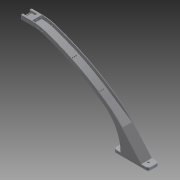
# Autodesk Inventor part: Lickport_Holder _v3
Saved by Autodesk Inventor 2012 SP2 (Build 160219200, 219)
## iProperties
Created: 2015-03-09
Part Number: Lickport_Holder _v3
Material: Default
Document SubType Name: Modeling
Designer: zhaox11
Density: 1 g/cm^3
Author: zhaox11
Autodesk Inventor part; units mm, degrees
ref_plane "YZ Plane" through (0, 0, 0) normal (1, 0, 0) x (0, 1, 0)
ref_plane "XZ Plane" through (0, 0, 0) normal (0, 1, 0) x (-1, 0, 0)
sketch "Sketch1" plane through (0, 0, 0) normal (0, 0, 1) x (1, 0, 0)
  line L0 (-50.8, 9.525) -> (-25.4, 9.525)
  line L1 (-25.4, 9.525) -> (-25.4, 0)
  line L2 (-25.4, 0) -> (-50.8, 0)
  line L3 (-50.8, 0) -> (-50.8, 9.525)
  line L4 (-25.4, -92.075) -> (11.1056, 20.2776)
  arc A0 (5.9961, 4.5523) -> (-25.4, 9.525) centre (-25.4, -92.075) ccw
  arc A1 (3.0527, -4.5065) -> (-25.4, 0) centre (-25.4, -92.075) ccw
  line L5 (-25.4, -92.075) -> (-197.4001, -621.4369)
  line L6 (-158.1658, -500.6861) -> (150.3246, -68.1948)
  arc A2 (150.3246, -68.1948) -> (5.9961, 4.5523) centre (-158.1658, -500.6861) ccw
  line L7 (150.3246, -68.1948) -> (159.8241, -54.8769)
  arc A3 (144.7934, -75.9493) -> (3.0527, -4.5065) centre (-158.1658, -500.6861) ccw
  line L8 (150.3246, -68.1948) -> (144.7934, -75.9493)
  line L9 (307.5871, -155.575) -> (-197.4001, -155.575)
  arc A4 (223.3152, -155.575) -> (150.3246, -68.1948) centre (19.4204, -251.7174) ccw
  arc A5 (212.7322, -155.575) -> (144.7934, -75.9493) centre (19.4204, -251.7174) ccw
  arc A6 (185.8036, -155.575) -> (144.7934, -75.9493) centre (87.9975, -155.575) ccw
  line L10 (87.9975, -155.575) -> (238.9402, -77.834)
  line L11 (189.2177, -103.4429) -> (19.4204, -251.7174)
  line L12 (189.2177, -103.4429) -> (234.7417, -155.575)
  line L13 (185.8036, -155.575) -> (212.7322, -155.575)
  line L14 (223.3152, -155.575) -> (212.7322, -155.575)
  line L15 (223.3152, -155.575) -> (234.7417, -155.575)
  line L16 (150.3246, -68.1948) -> (175.5181, -86.165)
  line L17 (145.7153, -74.6569) -> (144.7934, -75.9493)
  line L18 (144.7934, -75.9493) -> (145.7153, -74.6569)
  line L19 (145.7153, -74.6569) -> (189.2177, -103.4429)
  line L20 (234.7417, -155.575) -> (212.7322, -155.575)
  arc A7 (187.3911, -155.575) -> (145.7153, -74.6569) centre (87.9975, -155.575) ccw
  line L21 (187.3911, -155.575) -> (234.7417, -155.575)
  line L22 (145.7153, -74.6569) -> (150.3246, -68.1948)
  line L23 (234.7417, -155.575) -> (252.6778, -176.1147)
  point P0 (0, 0)
  dimension "d0" = 0
  dimension "d1" = 25.4
  dimension "d2" = 25.4
  dimension "d3" = 9.525
  dimension "d5" = 101.6
  dimension "d6" = 0
  dimension "d7" = 18
  dimension "d8" = 107.3658
  dimension "d29" = 17.5
  dimension "d55" = 165.1
  dimension "d56" = 54.5
  dimension "d57" = 27.25
  dimension "d70" = 7.9375
  constraints: 48 end point, 17 point on circle, 13 point on line, 10 collinear, 9 coincident, 8 centre point, 5 perpendicular, 2 parallel, 1 horizontal
  measures "d0" distance from line of point (0, 0) L2
  measures "d1" distance of L0.start L0.end
  measures "d2" distance from line of point (0, 0) L1
  measures "d3" distance of L2.end L0.start
  measures "d5" distance from line of L0 L4.start
  measures "d6" distance from line of L4.start L1
  measures "d7" angle of L4 L1
  measures "d8" distance from line of point (-158.166, -500.686) L3
  measures "d29" angle of L6 L5
  measures "d55" distance between parallel lines of L9 L0
  measures "d56" angle of L9 L6
  measures "d57" angle of L10 L6
  measures "d70" distance from line of L16 L17.start
extrude "Extrusion9" add sketch "Sketch1" against normal blind 25.4 contours L0 L1 L2 L3 | A0 L4 A1 L1 | A2 L6 A3 L4 | A4 L19 L6 | L6 A7 A5 | A5 A7 L10 A6 | L19 L10 A5 A7 | L12 L9 A4 | L11 A5 L10 | A4 L9 A5 L11 | A5 L10 A7 | L10 A7 L11 A6 | A5 L11 A7 L10 | A5 L9 A7 L11 | L11 A7 L9 A6
sketch "Sketch8" plane through (0, 0, 0) normal (0, 0, 1) x (1, 0, 0)
  line L0 (234.7417, -155.575) -> (185.8036, -155.575)
  line L1 (185.8036, -155.575) -> (185.8036, -161.925)
  line L2 (185.8036, -161.925) -> (234.7417, -161.925)
  line L3 (234.7417, -161.925) -> (234.7417, -155.575)
  point P0 (0, 0)
  dimension "d61" = 6.35
  constraints: 8 end point, 2 parallel, 1 horizontal, 1 perpendicular
  measures "d61" distance of L0.end L1.end
extrude "Extrusion10" add sketch "Sketch8" against normal blind 25.4
sketch "Sketch9" plane through (-50.8, 0, 0) normal (-1, 0, 0) x (0, 0, 1)
  line L0 (-25.4, 9.525) -> (-25.4, 0) projected
  line L1 (0, 0) -> (-25.4, 0) projected
  line L2 (0, 9.525) -> (0, 0) projected
  line L3 (0, 9.525) -> (-25.4, 9.525) projected
  line L4 (-23.8125, 9.525) -> (-1.5875, 9.525)
  line L5 (-1.5875, 9.525) -> (-1.5875, 1.5875)
  line L6 (-1.5875, 1.5875) -> (-23.8125, 1.5875)
  line L7 (-23.8125, 1.5875) -> (-23.8125, 9.525)
  dimension "d64" = 1.5875
  dimension "d65" = 1.5875
  dimension "d66" = 1.5875
  constraints: 8 end point, 2 parallel, 1 horizontal, 1 perpendicular, 1 point on line
  measures "d64" distance between parallel lines of L1 L6
  measures "d65" distance between parallel lines of L2 L5
  measures "d66" distance between parallel lines of L0 L7
sketch3d "3D Sketch2"
  line L0 (-50.8, 9.525, 0) -> (-25.4, 9.525, 0)
  arc A0 (-25.4, 9.525, 0) -> (5.9961, 4.5523, 0) centre (-25.4, -92.075, 0) ccw
  arc A1 (5.9961, 4.5523, 0) -> (150.3246, -68.1948, 0) centre (-158.1658, -500.6861, 0) ccw
  arc A2 (150.3246, -68.1948, 0) -> (189.2177, -103.4429, 0) centre (19.4204, -251.7174, 0) ccw
  line L1 (189.2177, -103.4429, 0) -> (234.7417, -155.575, 0)
sweep "Sweep2" cut profiles "Sketch9" path "3D Sketch2" contours L3 L5 L6 L7
sketch "Sketch13" plane through (228.7629, -160.7959, -1.5875) normal (-0.6577551, 0.7532319, 0) x (0.7532319, 0.6577551, 0)
  line L0 (0, 22.225) -> (0, 0) projected
  line L1 (0, 0) -> (7.9375, 0) projected
  line L2 (0, 22.225) -> (7.9375, 22.225)
  line L3 (7.9375, 22.225) -> (7.9375, 0)
  line L4 (7.9375, 0) -> (0, 0)
  line L5 (0, 0) -> (0, 22.225)
  point P0 (-66.5472, -1.5875)
  constraints: 8 end point, 2 parallel, 1 horizontal, 1 perpendicular
extrude "Extrusion14" cut sketch "Sketch13" against normal blind 25.4
extrude "Extrusion15" add sketch "Sketch1" against normal blind 25.4 contours L19 L10 A5 A7 | L12 L9 A4 | L11 A5 L10 | A4 L9 A5 L11 | A5 L10 A7 | A5 L11 A7 L10 | A5 L9 A7 L11
sketch "Sketch14" plane through (224.2038, -155.575, -1.5875) normal (0, -1, 0) x (1, 0, 0)
  line L0 (0, 0) -> (10.5379, 0)
  line L1 (10.5379, 0) -> (10.5379, -22.225)
  line L2 (10.5379, -22.225) -> (0, -22.225)
  line L3 (0, -22.225) -> (0, 0)
  point P0 (-224.2038, 1.5875)
  constraints: 8 end point, 2 parallel, 1 horizontal, 1 perpendicular
extrude "Extrusion16" add sketch "Sketch14" along normal blind 6.35
sketch "Sketch17" plane through (-50.8, 1.5875, -1.5875) normal (0, 1, 0) x (1, 0, 0)
  line L0 (0, 0) -> (25.4, 0) projected
  line L1 (25.4, 22.225) -> (17.78, 22.225)
  line L2 (17.78, 22.225) -> (17.78, 0)
  line L3 (17.78, 0) -> (25.4, 0)
  line L4 (25.4, 0) -> (25.4, 22.225)
  point P0 (50.8, -1.5875)
  dimension "d99" = 7.62
  constraints: 8 end point, 2 parallel, 1 horizontal, 1 perpendicular, 1 point on line
  measures "d99" distance of L1.start L1.end
extrude "Extrusion19" add sketch "Sketch17" along normal blind 7.9375
sketch "Sketch19" plane through (-25.4, 1.5875, -1.5875) normal (1, 0, 0) x (0, 0, -1)
  line L0 (22.225, 7.9375) -> (0, 7.9375) projected
  line L1 (22.225, 0) -> (0, 0) projected
  circle A0 centre (11.1125, 4.3942) radius 1.143
  line L2 (23.8125, 7.9375) -> (23.8125, 2.9648) projected
  circle A1 centre (11.1125, 1.143) radius 1.143
  circle A2 centre (1.143, 4.3942) radius 1.143
  circle A3 centre (21.082, 4.3942) radius 1.143
  line L3 (0, 7.9375) -> (0, 2.9648) projected
  line L4 (22.225, 2.9648) -> (22.225, 7.9375) projected
  line L5 (22.225, 7.9375) -> (22.225, 0) projected
  line L6 (21.082, 5.5372) -> (21.082, 4.3942)
  point P0 (-1.5875, -1.5875)
  dimension "d109" = 2.286
  dimension "d102" = 2.286
  dimension "d103" = 4.3942
  dimension "d104" = 7.9375
  dimension "d106" = 12.7
  dimension "d107" = 2.286
  dimension "d108" = 2.286
  dimension "d110" = 4.3942
  dimension "d111" = 4.3942
  dimension "d127" = 2.4003
  constraints: 3 centre point, 2 end point, 2 tangent, 1 coincident, 1 parallel, 1 vertical, 1 vertical alignment, 2 other
  measures "d102" diameter of A0
  measures "d103" distance from line of L1 A0.centre
  measures "d104" distance between parallel lines of L1 L0
  measures "d106" distance from line of L2 A0.centre
  measures "d107" diameter of A1
  measures "d108" diameter of A2
  measures "d110" distance from line of L1 A2.centre
  measures "d111" distance from line of L1 L6.end
  measures "d127" distance from line of L6.start L0
extrude "Extrusion20" cut sketch "Sketch19" against normal blind 7.62
sketch "Sketch20" plane through (-50.8, 1.5875, -1.5875) normal (0, 1, 0) x (1, 0, 0)
  line L0 (0, 0) -> (17.78, 0) projected
  line L1 (0, 22.225) -> (1.5875, 22.225)
  line L2 (1.5875, 22.225) -> (1.5875, 0)
  line L3 (1.5875, 0) -> (0, 0)
  line L4 (0, 0) -> (0, 22.225)
  point P0 (50.8, -1.5875)
  dimension "d114" = 1.5875
  constraints: 8 end point, 2 parallel, 1 horizontal, 1 perpendicular, 1 point on line
  measures "d114" distance between parallel lines of L2 L4
extrude "Extrusion21" add sketch "Sketch20" along normal blind 1.5875
sketch "Sketch21" plane through (-50.8, 3.175, -1.5875) normal (0, 1, 0) x (1, 0, 0)
  line L0 (1.5875, 22.225) -> (1.5875, 0) projected
  line L1 (0, 22.225) -> (1.5875, 22.225)
  line L2 (1.5875, 22.225) -> (1.5875, 19.05)
  line L3 (1.5875, 19.05) -> (0, 19.05)
  line L4 (0, 19.05) -> (0, 22.225)
  line L5 (0, 0) -> (1.5875, 0)
  line L6 (1.5875, 0) -> (1.5875, 3.175)
  line L7 (1.5875, 3.175) -> (0, 3.175)
  line L8 (0, 3.175) -> (0, 0)
  point P0 (50.8, -1.5875)
  dimension "d117" = 3.175
  dimension "d118" = 3.175
  constraints: 16 end point, 4 parallel, 2 horizontal, 2 perpendicular, 2 point on line
  measures "d117" distance of L3.end L1.start
  measures "d118" distance of L7.end L5.start
extrude "Extrusion22" add sketch "Sketch21" along normal blind 6.35
sketch "Sketch22" plane through (-33.02, 1.5875, -23.8125) normal (0, 0, 1) x (1, 0, 0)
  line L0 (0, 4.3942) -> (0, 7.9375) projected
  line L1 (-16.1925, 7.9375) -> (0, 7.9375) projected
  line L2 (-16.1925, 7.9375) -> (0, 7.9375)
  line L3 (0, 7.9375) -> (0, 6.35)
  line L4 (0, 6.35) -> (-16.1925, 6.35)
  line L5 (-16.1925, 6.35) -> (-16.1925, 7.9375)
  point P0 (33.02, -1.5875)
  dimension "d121" = 1.5875
  constraints: 8 end point, 2 parallel, 1 horizontal, 1 perpendicular, 1 point on line
  measures "d121" distance between parallel lines of L4 L2
extrude "Extrusion23" add sketch "Sketch22" along normal blind 3.175
sketch "Sketch23" plane through (-33.02, 5.9817, -1.5875) normal (0, 0, -1) x (-1, 0, 0)
  line L0 (16.1925, -4.3942) -> (16.1925, 3.5433) projected
  line L1 (0, 3.5433) -> (16.1925, 3.5433)
  line L2 (16.1925, 3.5433) -> (16.1925, 1.9558)
  line L3 (16.1925, 1.9558) -> (0, 1.9558)
  line L4 (0, 1.9558) -> (0, 3.5433)
  point P0 (-33.02, -5.9817)
  dimension "d124" = 1.5875
  constraints: 8 end point, 2 parallel, 1 horizontal, 1 perpendicular, 1 point on line
  measures "d124" distance between parallel lines of L3 L1
extrude "Extrusion24" add sketch "Sketch23" along normal blind 3.175
sketch "Sketch24" plane through (0, 0, 0) normal (0, 0, 1) x (1, 0, 0)
  circle A0 centre (-10.4817, 2.1152) radius 1.27
  arc A1 (5.9961, 4.5523) -> (-25.4, 9.525) centre (-25.4, -92.075) ccw projected
  line L0 (-50.8, 0) -> (-25.4, 0) projected
  arc A2 (3.0527, -4.5065) -> (-25.4, 0) centre (-25.4, -92.075) ccw projected
  line L1 (234.7417, -161.925) -> (234.7417, -155.575) projected
  line L2 (-25.4, -92.075) -> (-7.073, 23.6369)
  line L3 (-25.4, -92.075) -> (-25.4, 0)
  line L4 (-10.4817, 2.1152) -> (-5.7845, 1.3712)
  line L5 (-25.4, -92.075) -> (-0.7179, 0.0398)
  line L6 (-0.7179, 0.0398) -> (6.1959, -1.8127)
  circle A3 centre (-0.7179, 0.0398) radius 1.27
  point P0 (0, 0)
  dimension "d128" = 2.54
  dimension "d134" = 9
  dimension "d135" = 92.075
  dimension "d136" = 95.3643
  dimension "d137" = 14.9183
  dimension "d138" = 2.1152
  dimension "d139" = 6
  dimension "d140" = 95.3643
  dimension "d141" = 2.54
  constraints: 10 end point, 2 centre point, 2 coincident, 2 perpendicular, 1 parallel, 1 point on line
  measures "d128" diameter of A0
  measures "d134" angle of L2 L3
  measures "d135" distance of L2.start L0.end
  measures "d136" distance from line of A1.centre L4
  measures "d137" distance from line of L3 A0.centre
  measures "d138" distance from line of L0 A0.centre
  measures "d139" angle of L5 L2
  measures "d140" distance from line of A1.centre L6
  measures "d141" diameter of A3
extrude "Extrusion26" cut sketch "Sketch24" against normal blind 25.4 contours A0 L4 L2 | L2 A0 | A0 L2 L4 | A3 L6 L5 | L5 L6 A3
sketch "Sketch25" plane through (185.8036, -161.925, 0) normal (-1, 0, 0) x (0, 0, 1)
  line L0 (-25.4, 6.35) -> (-25.4, 0) projected
  line L1 (0, 0) -> (-25.4, 0) projected
  line L2 (-25.4, 6.35) -> (0, 6.35)
  line L3 (0, 6.35) -> (0, 0)
  line L4 (0, 0) -> (-25.4, 0)
  line L5 (-25.4, 0) -> (-25.4, 6.35)
  point P0 (0, 161.925)
  constraints: 8 end point, 2 parallel, 1 horizontal, 1 perpendicular
extrude "Extrusion27" add sketch "Sketch25" along normal blind 16.51
sketch "Sketch26" plane through (234.7417, -161.925, -25.4) normal (0, -1, 0) x (1, 0, 0)
  line L0 (0, 25.4) -> (0, 0) projected
  line L1 (-65.4481, 25.4) -> (0, 25.4) projected
  line L2 (-65.4481, 25.4) -> (-65.4481, 0) projected
  line L3 (-65.4481, 0) -> (0, 0) projected
  line L4 (-65.4481, 25.4) -> (17.1019, 25.4)
  line L5 (17.1019, 25.4) -> (17.1019, 0)
  line L6 (17.1019, 0) -> (-65.4481, 0)
  line L7 (-65.4481, 0) -> (-65.4481, 25.4)
  circle A0 centre (4.4019, 12.7) radius 2.286
  circle A1 centre (-55.9231, 12.7) radius 2.286
  point P0 (-234.7417, 25.4)
  dimension "d146" = 82.55
  dimension "d149" = 4.572
  dimension "d150" = 12.7
  dimension "d151" = 4.572
  dimension "d152" = 60.325
  constraints: 8 end point, 2 centre point, 2 parallel, 1 horizontal, 1 perpendicular
  measures "d146" distance of L5.end L6.end
  measures "d149" diameter of A0
  measures "d150" distance from line of L5 A0.centre
  measures "d151" diameter of A1
  measures "d152" distance of A0.centre A1.centre
extrude "Extrusion28" add sketch "Sketch26" against normal blind 6.35 contours L4 L5 L6 L0 | A0
extrude "Extrusion29" cut sketch "Sketch26" against normal blind 6.35 contours A0 | A1
fillet "Fillet2" radius 6.35 4 edges at (169.2936, -158.75, 0) (251.8436, -158.75, 0) (251.8436, -158.75, -25.4) (169.2936, -158.75, -25.4)
sketch "Sketch27" plane through (0, 0, -25.4) normal (0, 0, -1) x (-1, 0, 0)
  line L0 (-175.6436, -155.575) -> (-175.6436, -161.925) projected
  line L1 (-185.8036, -155.575) -> (-175.6436, -155.575) projected
  arc A0 (-144.7934, -75.9493) -> (-185.8036, -155.575) centre (-87.9975, -155.575) ccw projected
  arc A1 (-3.0527, -4.5065) -> (-144.7934, -75.9493) centre (158.1658, -500.6861) ccw projected
  arc A2 (25.4, 0) -> (-3.0527, -4.5065) centre (25.4, -92.075) ccw projected
  line L2 (50.8, 0) -> (25.4, 0) projected
  line L3 (50.8, 9.525) -> (50.8, 0) projected
  line L4 (25.4, 9.525) -> (50.8, 9.525) projected
  arc A3 (25.4, 9.525) -> (-5.9961, 4.5523) centre (25.4, -92.075) ccw projected
  arc A4 (-5.9961, 4.5523) -> (-150.3246, -68.1948) centre (158.1658, -500.6861) ccw projected
  arc A5 (-150.3246, -68.1948) -> (-189.2177, -103.4429) centre (-19.4204, -251.7174) ccw projected
  line L5 (-234.7417, -155.575) -> (-189.2177, -103.4429) projected
  line L6 (-234.7417, -155.575) -> (-245.4936, -155.575) projected
  line L7 (-245.4936, -161.925) -> (-245.4936, -155.575) projected
  line L8 (-175.6436, -161.925) -> (-245.4936, -161.925) projected
  circle A6 centre (0.7179, 0.0398) radius 1.27 projected
  circle A7 centre (10.4817, 2.1152) radius 1.27 projected
  line L9 (-251.8436, -155.575) -> (-251.8436, -161.925) projected
  point P0 (0, 0)
  dimension "d156" = 302.6436
  dimension "d157" = 171.45
  measures "d156" distance between parallel lines of L9 L3
  measures "d157" distance between parallel lines of L4 L8
sketch "Sketch28" plane through (0, 0, 0) normal (0, 0, 1) x (1, 0, 0)
  line L0 (245.4936, -155.575) -> (245.4936, -161.925) projected
  line L1 (245.4936, -155.575) -> (234.7417, -155.575) projected
  line L2 (234.7417, -155.575) -> (189.2177, -103.4429) projected
  arc A0 (189.2177, -103.4429) -> (150.3246, -68.1948) centre (19.4204, -251.7174) ccw projected
  arc A1 (150.3246, -68.1948) -> (5.9961, 4.5523) centre (-158.1658, -500.6861) ccw projected
  arc A2 (5.9961, 4.5523) -> (-25.4, 9.525) centre (-25.4, -92.075) ccw projected
  line L3 (-25.4, 9.525) -> (-50.8, 9.525) projected
  line L4 (-50.8, 9.525) -> (-50.8, 0) projected
  line L5 (-50.8, 0) -> (-25.4, 0) projected
  arc A3 (3.0527, -4.5065) -> (-25.4, 0) centre (-25.4, -92.075) ccw projected
  arc A4 (144.7934, -75.9493) -> (3.0527, -4.5065) centre (-158.1658, -500.6861) ccw projected
  arc A5 (185.8036, -155.575) -> (144.7934, -75.9493) centre (87.9975, -155.575) ccw projected
  line L6 (185.8036, -155.575) -> (175.6436, -155.575) projected
  line L7 (175.6436, -161.925) -> (175.6436, -155.575) projected
  line L8 (175.6436, -161.925) -> (245.4936, -161.925) projected
  circle A6 centre (-0.7179, 0.0398) radius 1.27 projected
  circle A7 centre (-10.4817, 2.1152) radius 1.27 projected
  line L9 (-69.3284, 44.0459) -> (254.3206, -106.8742)
  point P0 (0, 0)
  point P1 (66.3456, -19.2199)
  dimension "d158" = 25
  constraints: 2 end point, 1 point on circle, 1 point on line, 1 tangent
  measures "d158" angle of L5 L9
sketch "Sketch29" plane through (0, 0, -25.4) normal (0, 0, -1) x (-1, 0, 0)
  line L0 (-175.6436, -155.575) -> (-175.6436, -161.925) projected
  line L1 (-185.8036, -155.575) -> (-175.6436, -155.575) projected
  arc A0 (-144.7934, -75.9493) -> (-185.8036, -155.575) centre (-87.9975, -155.575) ccw projected
  arc A1 (-3.0527, -4.5065) -> (-144.7934, -75.9493) centre (158.1658, -500.6861) ccw projected
  arc A2 (25.4, 0) -> (-3.0527, -4.5065) centre (25.4, -92.075) ccw projected
  line L2 (50.8, 0) -> (25.4, 0) projected
  line L3 (50.8, 9.525) -> (50.8, 0) projected
  line L4 (25.4, 9.525) -> (50.8, 9.525) projected
  arc A3 (25.4, 9.525) -> (-5.9961, 4.5523) centre (25.4, -92.075) ccw projected
  arc A4 (-5.9961, 4.5523) -> (-150.3246, -68.1948) centre (158.1658, -500.6861) ccw projected
  arc A5 (-150.3246, -68.1948) -> (-189.2177, -103.4429) centre (-19.4204, -251.7174) ccw projected
  line L5 (-234.7417, -155.575) -> (-189.2177, -103.4429) projected
  line L6 (-234.7417, -155.575) -> (-245.4936, -155.575) projected
  line L7 (-245.4936, -161.925) -> (-245.4936, -155.575) projected
  line L8 (-175.6436, -161.925) -> (-245.4936, -161.925) projected
  circle A6 centre (0.7179, 0.0398) radius 1.27 projected
  circle A7 centre (10.4817, 2.1152) radius 1.27 projected
  line L9 (66.7155, 42.8275) -> (-222.1048, -91.8517)
  point P0 (0, 0)
  point P1 (-66.3456, -19.2199)
  dimension "d159" = 25
  constraints: 2 end point, 1 point on circle, 1 point on line, 1 tangent
  measures "d159" angle of L2 L9
sketch3d "3D Sketch3"
ref_plane "Work Plane3" through (-69.3284, 44.0459, 0) normal (0.4226183, 0.9063078, 0) x (0.9063078, -0.4226183, 0)
sketch "Sketch31" plane through (-69.3284, 44.0459, 0) normal (0.4226183, 0.9063078, 0) x (0.9063078, -0.4226183, 0)
  circle A0 centre (149.7694, 8.382) radius 1.397
  line L0 (84.9579, 0) -> (246.5082, 0) projected
  circle A1 centre (149.7694, 17.018) radius 1.397
  line L1 (84.9579, 25.4) -> (246.5082, 25.4) projected
  circle A2 centre (149.7694, 12.7) radius 1.397
  point P0 (81.4474, 0)
  dimension "d160" = 2.794
  dimension "d161" = 8.382
  dimension "d162" = 2.794
  dimension "d163" = 8.382
  dimension "d173" = 2.794
  dimension "d174" = 8.636
  dimension "d175" = 4.318
  constraints: 3 centre point
  measures "d160" diameter of A0
  measures "d161" distance from line of L0 A0.centre
  measures "d162" diameter of A1
  measures "d163" distance from line of A1.centre L1
  measures "d173" diameter of A2
  measures "d174" distance of A0.centre A1.centre
  measures "d175" distance of A2.centre A1.centre
sketch "Sketch32" plane through (-69.3284, 44.0459, 0) normal (0.4226183, 0.9063078, 0) x (0.9063078, -0.4226183, 0)
  circle A0 centre (224.2034, 17.018) radius 1.397
  circle A1 centre (224.2034, 8.382) radius 1.397
  line L0 (84.9579, 25.4) -> (246.5082, 25.4) projected
  line L1 (84.9579, 0) -> (246.5082, 0) projected
  circle A2 centre (224.2034, 12.7) radius 1.397
  point P0 (81.4474, 0)
  dimension "d166" = 2.794
  dimension "d167" = 2.794
  dimension "d168" = 8.382
  dimension "d169" = 8.382
  dimension "d170" = 0
  dimension "d176" = 2.794
  dimension "d177" = 8.636
  dimension "d178" = 4.318
  constraints: 3 centre point
  measures "d166" diameter of A0
  measures "d167" diameter of A1
  measures "d168" distance from line of L0 A0.centre
  measures "d169" distance from line of L1 A1.centre
  measures "d170" horizontal distance of A1.centre A0.centre
  measures "d176" diameter of A2
  measures "d177" distance of A1.centre A0.centre
  measures "d178" distance of A0.centre A2.centre
extrude "Extrusion32" cut sketch "Sketch31" against normal blind 38.1
extrude "Extrusion33" cut sketch "Sketch32" against normal blind 38.1
equation "\"d57\" = 0.5 * d56"
equation "\"d110\" = d103"
equation "\"d111\" = d103"
equation "\"d140\" = d136"
body "Solid5"
